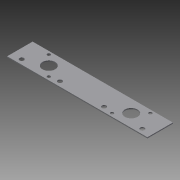
# Autodesk Inventor part: launcher_connector
Saved by Autodesk Inventor 2013 (Build 170138000, 138)
## iProperties
Created: 2013-07-25
Part Number: launcher_connector
Material: Generic
Document SubType Name: Modeling
Designer: dkboone
Density: 1 g/cm^3
Author: dkboone
Autodesk Inventor part; units mm, degrees
ref_plane "YZ Plane" through (0, 0, 0) normal (1, 0, 0) x (0, 1, 0)
ref_plane "XZ Plane" through (0, 0, 0) normal (0, 1, 0) x (-1, 0, 0)
ref_plane "XY Plane" through (0, 0, 0) normal (0, 0, 1) x (1, 0, 0)
sketch "Sketch1" plane through (0, 0, 0) normal (0, 1, 0) x (-1, 0, 0)
  line L0 (-69.85, 25.4) -> (69.85, 25.4)
  line L1 (69.85, 25.4) -> (69.85, 0)
  line L2 (69.85, 0) -> (-69.85, 0)
  line L3 (-69.85, 0) -> (-69.85, 25.4)
  circle A0 centre (-41.021, 12.7) radius 6.35
  circle A1 centre (-31.496, 22.225) radius 1.5875
  circle A2 centre (-50.546, 3.175) radius 1.5875
  line L4 (-53.721, 25.4) -> (-53.721, 0) construction
  line L5 (53.721, 25.4) -> (53.721, 0) construction
  line L6 (-28.321, 25.4) -> (-28.321, 0) construction
  line L7 (28.321, 25.4) -> (28.321, 0) construction
  line L8 (0, 0) -> (0, 25.4) construction
  circle A3 centre (41.021, 12.7) radius 6.35
  circle A4 centre (31.496, 22.225) radius 1.5875
  circle A5 centre (50.546, 3.175) radius 1.5875
  circle A6 centre (-60.071, 20.6375) radius 2.1526
  circle A7 centre (-21.971, 20.6375) radius 2.1526
  circle A8 centre (60.071, 20.6375) radius 2.1526
  circle A9 centre (21.971, 20.6375) radius 2.1526
  dimension "d0" = 139.7
  dimension "d2" = 69.85
  dimension "d3" = 25.4
  dimension "d4" = 12.7
  dimension "d5" = 3.175
  dimension "d6" = 3.175
  dimension "d7" = 107.442
  dimension "d8" = 16.129
  dimension "d9" = 3.175
  dimension "d10" = 3.175
  dimension "d11" = 25.4
  dimension "d12" = 25.4
  dimension "d13" = 3.175
  dimension "d14" = 3.175
  dimension "d15" = 12.7
  dimension "d16" = 12.7
  dimension "d17" = 4.3053
  dimension "d18" = 4.3053
  dimension "d19" = 4.7625
  dimension "d20" = 4.7625
  dimension "d21" = 6.35
  dimension "d22" = 6.35
  constraints: 18 end point, 10 centre point, 8 point on line, 5 perpendicular, 5 symmetric about line, 2 midpoint, 2 parallel, 1 horizontal, 5 other
  measures "d0" distance of L0.start L0.end
  measures "d2" distance from line of L1 L8.start
  measures "d3" distance of L2.end L0.start
  measures "d4" diameter of A0
  measures "d5" diameter of A1
  measures "d6" diameter of A2
  measures "d7" distance between parallel lines of L5 L4
  measures "d8" distance between parallel lines of L1 L5
  measures "d9" distance from line of A2.centre L4
  measures "d10" distance from line of L2 A2.centre
  measures "d11" distance between parallel lines of L6 L4
  measures "d12" distance between parallel lines of L5 L7
  measures "d13" distance from line of L6 A1.centre
  measures "d14" distance from line of L0 A1.centre
  measures "d15" distance from line of L2 A0.centre
  measures "d16" distance from line of L6 A0.centre
  measures "d17" diameter of A6
  measures "d18" diameter of A7
  measures "d19" distance from line of L0 A6.centre
  measures "d20" distance from line of L0 A7.centre
  measures "d21" distance from line of L6 A7.centre
  measures "d22" distance from line of L4 A6.centre
extrude "Extrusion1" add sketch "Sketch1" along normal blind 1.016
equation "\"d2\" = 0.5 * d0"
equation "\"d8\" = -0.5 * d7 + 0.5 * d0"
body "Solid1"
